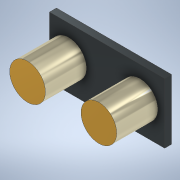
# Autodesk Inventor part: Ultrasonic Sensor
Saved by Autodesk Inventor 2021 (Build 250183000, 183)
## iProperties
Created: 2021-06-27
Part Number: Ultrasonic Sensor
Material: Generic
Document SubType Name: Modeling
Designer: ShivAni
Density: 1 g/cm^3
Appearance: Default
Author: ShivAni
Autodesk Inventor part; units mm, degrees
ref_plane "YZ Plane" through (0, 0, 0) normal (1, 0, 0) x (0, 1, 0)
ref_plane "XZ Plane" through (0, 0, 0) normal (0, 1, 0) x (-1, 0, 0)
ref_plane "XY Plane" through (0, 0, 0) normal (0, 0, 1) x (1, 0, 0)
sketch "Sketch1" plane through (0, 0, 0) normal (0, 0, 1) x (1, 0, 0)
  point P0 (0, 0)
sketch "Sketch2" plane through (0, 0, 0) normal (0, 0, 1) x (1, 0, 0)
  line L0 (0, 0) -> (42, 0)
  line L1 (42, 0) -> (42, 22)
  line L2 (42, 22) -> (0, 22)
  line L3 (0, 22) -> (0, 0)
  dimension "d0" = 42
  dimension "d1" = 22
  constraints: 8 end point, 2 parallel, 1 horizontal, 1 perpendicular
  measures "d0" distance of L2.end L1.end
  measures "d1" distance of L1.end L0.end
extrude "Extrusion1" add sketch "Sketch2" along normal blind 2.54
sketch "Sketch3" plane through (0, 0, 2.54) normal (0, 0, 1) x (1, 0, 0)
  circle A0 centre (7, 11) radius 6.5
  circle A1 centre (33, 11) radius 6.5
  line L0 (0, 22) -> (0, 0) projected
  line L1 (42, 0) -> (42, 22) projected
  dimension "d4" = 13
  dimension "d5" = 13
  dimension "d6" = 7
  dimension "d7" = 9
  constraints: 2 centre point
  measures "d4" diameter of A0
  measures "d5" diameter of A1
  measures "d6" distance from line of L0 A0.centre
  measures "d7" distance from line of L1 A1.centre
extrude "Extrusion2" add sketch "Sketch3" along normal blind 15
body "Solid1"
